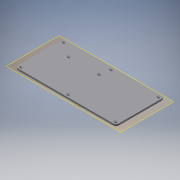
# Autodesk Inventor part: bottom
Saved by Autodesk Inventor 2017.3 (Build 213257000, 257)
## iProperties
Created: 2021-12-05
Part Number: bottom
Material: Generic
Document SubType Name: Modeling
Designer: TEOS
Density: 1 g/cm^3
Appearance: Default
Author: TEOS
Autodesk Inventor part; units mm, degrees
ref_plane "YZ Plane" through (0, 0, 0) normal (1, 0, 0) x (0, 1, 0)
ref_plane "XZ Plane" through (0, 0, 0) normal (0, 1, 0) x (-1, 0, 0)
ref_plane "XY Plane" through (0, 0, 0) normal (0, 0, 1) x (1, 0, 0)
ref_plane "Work Plane1" through (0, 0, -3) normal (0, 0, 1) x (1, 0, 0)
sketch "Sketch2" plane through (0, 0, -3) normal (0, 0, 1) x (1, 0, 0)
  circle A0 centre (-82, -37) radius 1 projected
  circle A1 centre (0, -37) radius 1 projected
  circle A2 centre (82, 37) radius 1 projected
  circle A3 centre (0, 37) radius 1 projected
  circle A4 centre (82, -37) radius 1 projected
  circle A5 centre (-82, 37) radius 1 projected
  arc A6 (-77, -37) -> (-82, -32) centre (-82, -37) ccw projected
  line L0 (-82, -32) -> (-82, 32) projected
  arc A7 (-82, 32) -> (-77, 37) centre (-82, 37) ccw projected
  line L1 (-77, 37) -> (-5, 37) projected
  arc A8 (-5, 37) -> (5, 37) centre (0, 37) ccw projected
  line L2 (5, 37) -> (77, 37) projected
  arc A9 (77, 37) -> (82, 32) centre (82, 37) ccw projected
  line L3 (82, 32) -> (82, -32) projected
  arc A10 (82, -32) -> (77, -37) centre (82, -37) ccw projected
  line L4 (77, -37) -> (5, -37) projected
  arc A11 (5, -37) -> (-5, -37) centre (0, -37) ccw projected
  line L5 (-5, -37) -> (-77, -37) projected
  line L6 (82, -42) -> (-82, -42) projected
  arc A12 (82, -42) -> (87, -37) centre (82, -37) ccw projected
  line L7 (87, 37) -> (87, -37) projected
  arc A13 (87, 37) -> (82, 42) centre (82, 37) ccw projected
  line L8 (-82, 42) -> (82, 42) projected
  arc A14 (-82, 42) -> (-87, 37) centre (-82, 37) ccw projected
  line L9 (-87, -37) -> (-87, 37) projected
  arc A15 (-87, -37) -> (-82, -42) centre (-82, -37) ccw projected
  point P0 (0, 0)
extrude "Extrusion1" add sketch "Sketch2" along normal blind 3 contours A6 L0 A7 L1 A8 L2 A9 L3 A10 L4 A11 L5 | L6 A15 L9 A14 L8 A13 L7 A12
sketch "Sketch3" plane through (0, 0, 0) normal (0, 0, 1) x (1, 0, 0)
  circle A0 centre (-82, 37) radius 1 projected
  circle A1 centre (82, -37) radius 1 projected
  circle A2 centre (0, 37) radius 1 projected
  circle A3 centre (82, 37) radius 1 projected
  circle A4 centre (0, -37) radius 1 projected
  circle A5 centre (-82, -37) radius 1 projected
  line L0 (-82, -42) -> (82, -42) projected
  arc A6 (82, -42) -> (87, -37) centre (82, -37) ccw projected
  line L1 (87, -37) -> (87, 37) projected
  arc A7 (87, 37) -> (82, 42) centre (82, 37) ccw projected
  line L2 (82, 42) -> (-82, 42) projected
  arc A8 (-82, 42) -> (-87, 37) centre (-82, 37) ccw projected
  line L3 (-87, 37) -> (-87, -37) projected
  arc A9 (-87, -37) -> (-82, -42) centre (-82, -37) ccw projected
  circle A10 centre (-82, 37) radius 1 projected
  circle A11 centre (82, 37) radius 1 projected
  point P0 (0, 0)
  constraints: 6 coincident
hole "Hole1" at (82, -37, 0) at (0, -37, 0) at (-82, -37, 0) at (-82, 37, 0) at (0, 37, 0) at (82, 37, 0) direction (0, 0, -1) diameter 3 depth 15 tip angle 118 countersink diameter 6 countersink angle 90
sketch "Sketch9" plane through (0, 0, -3) normal (0, 0, -1) x (-1, 0, 0)
  circle A0 centre (-28.4857, -17.7776) radius 1.5 projected
  circle A1 centre (-75.4853, -20.7832) radius 1.5 projected
  circle A2 centre (-62.2844, 31.2184) radius 1.5 projected
  circle A3 centre (-30.6986, 31.2222) radius 1.5 projected
  circle A4 centre (-28.4857, -17.7776) radius 3
  circle A5 centre (-75.4853, -20.7832) radius 3
  circle A6 centre (-30.6986, 31.2222) radius 3
  circle A7 centre (-62.2844, 31.2184) radius 3
  point P0 (0, 0)
  dimension "d38" = 6
  dimension "d39" = 6
  dimension "d40" = 6
  dimension "d41" = 6
  constraints: 4 centre point, 4 coincident
  measures "d38" diameter of A4
  measures "d39" diameter of A5
  measures "d40" diameter of A6
  measures "d41" diameter of A7
extrude "Extrusion4" add sketch "Sketch9" along normal blind 5 contours A0 | A1 | A2 | A3 | A4 | A5 | A6 | A7
sketch "Sketch10" plane through (28.4857, -17.7776, -8) normal (0, 0, -1) x (-1, 0, 0)
  circle A0 centre (0, 0) radius 3 projected
  circle A1 centre (-46.9996, -3.0056) radius 3 projected
  circle A2 centre (-33.7987, 48.996) radius 3 projected
  circle A3 centre (-2.2129, 48.9997) radius 3 projected
  point P0 (28.4857, 17.7776)
  point P1 (-2.2129, 48.9997)
  constraints: 4 coincident
hole "Hole2" at (28.4857, -17.7776, -8) at (30.6986, 31.2222, -8) at (62.2844, 31.2184, -8) at (75.4853, -20.7832, -8) direction (0, 0, 1) diameter 2 depth 5
sketch "Sketch16" plane through (0, 0, -3) normal (0, 0, -1) x (-1, 0, 0)
  circle A0 centre (-0.7595, -10.8276) radius 11.876 projected
  circle A1 centre (-0.7595, -10.8276) radius 13.5
  point P0 (0, 0)
  dimension "d78" = 27
  constraints: 1 centre point, 1 coincident
  measures "d78" diameter of A1
extrude "Extrusion9" add sketch "Sketch16" along normal blind 20 contours A0 | A1
thread "Thread3" size "M27x3" class "6g" standard "ISO Metric profile" full length
sketch "Sketch18" plane through (0.7595, -10.8276, -23) normal (1, 0, 0) x (0, 1, 0)
  line L0 (13.5, 0) -> (13.5, 20)
  line L1 (13.5, 20) -> (11.2756, 20)
  line L2 (11.2756, 20) -> (11.2756, 0)
  line L3 (11.2756, 0) -> (13.5, 0)
  line L4 (0, -9.4) -> (0, 28.4) projected
  constraints: 8 end point
revolve "Revolution3" cut sketch "Sketch18" angle 360 about axis through (0.7595, -10.8276, -23) along (0, 0, 1)
sketch "Sketch19" plane through (0.7595, -10.8276, -23) normal (1, 0, 0) x (0, 1, 0)
  line L0 (13.5, 0) -> (13.5, 20)
  line L1 (13.5, 20) -> (11.2756, 20)
  line L2 (11.2756, 20) -> (11.2756, 0)
  line L3 (11.2756, 0) -> (13.5, 0)
  line L4 (0, -9.4) -> (0, 28.4) projected
  constraints: 8 end point
revolve "Revolution4" add sketch "Sketch19" angle 360 about axis through (0.7595, -10.8276, -23) along (0, 0, 1) separate body
sketch "Sketch17" plane through (0.7595, -10.8276, -23) normal (-1, 0, 0) x (0, 0, 1)
  line L0 (-1.7501, -11.4275) -> (-1.5001, -11.4275) construction
  line L1 (0.2499, -13.3485) -> (-0.0001, -13.8287) construction
  line L2 (-3.0001, -13.8287) -> (-3.2501, -13.3485) construction
  line L3 (-1.2501, -11.4275) -> (-1.5001, -10.9472) construction
  line L4 (-1.5001, -10.9472) -> (-1.7501, -11.4275) construction
  line L5 (-3.0001, -13.8287) -> (-2.7501, -13.3485) construction
  line L6 (-1.2501, -11.4275) -> (-0.2501, -13.3485)
  line L7 (-3.2501, -13.3485) -> (-2.7501, -13.3485) construction
  arc A0 (-3.2501, -13.3485) -> (-3.0001, -13.5002) centre (-3.0001, -13.2183) ccw construction
  line L8 (0.2499, -13.3485) -> (-0.2501, -13.3485) construction
  line L9 (-3.0001, -13.8287) -> (-3.0001, -13.3485) construction
  line L10 (-0.0001, -13.8287) -> (-0.0001, -13.3485) construction
  line L11 (-1.5001, -10.9472) -> (-1.5001, -11.2758) construction
  line L12 (-3.0001, -13.5002) -> (-0.0001, -13.5002)
  arc A1 (-3.0001, -13.5002) -> (-2.7501, -13.3485) centre (-3.0001, -13.2183) ccw
  line L13 (-0.2501, -13.3485) -> (-0.0001, -13.8287) construction
  line L14 (-2.7501, -13.3485) -> (-1.7501, -11.4275)
  line L15 (-0.0001, -0.0002) -> (-0.0001, 0.0177)
  line L16 (-0.0001, 0.0177) -> (-0.0001, -0.0002)
  line L17 (-0.0001, -0.0002) -> (0.0334, -0.0002)
  arc A2 (-0.2501, -13.3485) -> (-0.0001, -13.5002) centre (-0.0001, -13.2183) ccw
  arc A3 (-0.0001, -13.5002) -> (0.2499, -13.3485) centre (-0.0001, -13.2183) ccw construction
  arc A4 (-1.5001, -11.2758) -> (-1.7501, -11.4275) centre (-1.5001, -11.5576) ccw
  arc A5 (-1.2501, -11.4275) -> (-1.5001, -11.2758) centre (-1.5001, -11.5576) ccw
  line L18 (-1.5001, -11.2758) -> (-1.5001, -11.4275) construction
  line L19 (-1.5001, -11.4275) -> (-1.2501, -11.4275) construction
  dimension "d83" = 55
  dimension "d84" = 0.4803
  dimension "d85" = 0.4803
  dimension "Sketch17_ThreadOffset" = 0
  dimension "Sketch17_MajorRadius" = 13.5
  dimension "d88" = 3
  dimension "Sketch17_MinorRadius" = 11.2756
  constraints: 40 end point, 12 point on circle, 10 parallel, 8 tangent, 6 centre point, 6 collinear, 2 midpoint, 2 point on line, 1 horizontal, 1 perpendicular, 3 other
  measures "d83" angle of L6 L14
  measures "d84" distance of L3.end L0.end
  measures "d85" distance of L1.end L10.end
  measures "Sketch17_ThreadOffset" distance between parallel lines of L15 L10
  measures "Sketch17_MajorRadius" distance from line of L12 L15.start
  measures "d88" distance from line of L1.end L9
  measures "Sketch17_MinorRadius" distance edge to line of A5 L17
coil "Coil2" sketch "Sketch17" operation cut axis through (0.7595, -10.8276, -23) along (0, 0, 1) pitch 3.003 turns 8.658009 hand right bodies 2
sketch "Sketch20" plane through (0, 0, 0) normal (0, 0, 1) x (1, 0, 0)
  circle A0 centre (-55.85, 19.5) radius 1 projected
  line L0 (-31, 9.5) -> (-31, 29.5) projected
  line L1 (-31, 9.5) -> (-79.2, 9.5) projected
  line L2 (-79.2, 29.5) -> (-79.2, 9.5) projected
  line L3 (-79.2, 29.5) -> (-31, 29.5) projected
  circle A1 centre (-3.15, 19.5) radius 1 projected
  line L4 (-28, 29.5) -> (-28, 9.5) projected
  line L5 (-28, 29.5) -> (20.2, 29.5) projected
  line L6 (20.2, 9.5) -> (20.2, 29.5) projected
  line L7 (20.2, 9.5) -> (-28, 9.5) projected
  point P0 (0, 0)
  constraints: 2 coincident
hole "Hole4" at (-55.85, 19.5, 0) at (-3.15, 19.5, 0) direction (0, 0, -1) diameter 3 end through all countersink diameter 6 countersink angle 90 bodies 1
equation "\"d83\" = d90"
equation "\"d84\" = 0.160083 * Sketch17_Pitch"
equation "\"d85\" = 0.160083 * Sketch17_Pitch"
equation "\"d88\" = Sketch17_Pitch"
equation "\"d26\" = 55deg"
equation "\"Sketch6_Pitch\" = 3"
equation "\"d90\" = 55deg"
equation "\"Sketch17_Pitch\" = 3"
body "Solid1"
body "Solid3"
